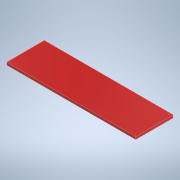
# Autodesk Inventor part: Hanging Platform
Saved by Autodesk Inventor 2021 (Build 250183000, 183)
## iProperties
Created: 2021-02-06
Part Number: Hanging Platform
Material: Rubber, Silicone
Document SubType Name: Modeling
Designer: aidan
Density: 1.25 g/cm^3
Appearance: Red
Author: aidan
Autodesk Inventor part; units mm, degrees
ref_plane "YZ Plane" through (0, 0, 0) normal (1, 0, 0) x (0, 1, 0)
ref_plane "XZ Plane" through (0, 0, 0) normal (0, 1, 0) x (-1, 0, 0)
ref_plane "XY Plane" through (0, 0, 0) normal (0, 0, 1) x (1, 0, 0)
sketch "Sketch1" plane through (0, 0, 0) normal (0, 1, 0) x (-1, 0, 0)
  line L0 (0, 0) -> (-3657.6, 0)
  line L1 (-3657.6, 0) -> (-3657.6, -1066.8)
  line L2 (-3657.6, -1066.8) -> (0, -1066.8)
  line L3 (0, -1066.8) -> (0, 0)
  dimension "d0" = 3657.6
  dimension "d1" = 1066.8
  constraints: 8 end point, 2 parallel, 1 horizontal, 1 perpendicular
  measures "d0" distance of L1.end L2.end
  measures "d1" distance of L0.end L1.end
extrude "Extrusion1" add sketch "Sketch1" along normal blind 76.2
sketch "Sketch2" plane through (0, 76.2, 0) normal (0, 1, 0) x (1, 0, 0)
  circle A0 centre (50.8, 50.8) radius 1.905
  line L0 (0, 0) -> (3657.6, 0) projected
  line L1 (0, 1066.8) -> (0, 0) projected
  line L2 (60.325, 63.6506) -> (60.325, 37.6088) construction
  dimension "d4" = 3.81
  dimension "d5" = 50.8
  dimension "d6" = 50.8
  dimension "d7" = 9.525
  constraints: 2 end point, 1 centre point, 1 vertical
  measures "d4" diameter of A0
  measures "d5" distance from line of L0 A0.centre
  measures "d6" distance from line of L1 A0.centre
  measures "d7" distance from line of L2 A0.centre
revolve "Revolution1" cut sketch "Sketch2" angle 180 about axis through (60.325, 76.2, -63.6506) along (0, 0, 1)
sketch "Sketch3" plane through (0, 76.2, 0) normal (0, 1, 0) x (1, 0, 0)
  circle A0 centre (50.8, 50.8) radius 1.905 projected
  line L0 (50.8, 50.8) -> (3597.275, 50.8) construction
  line L1 (3597.275, 50.8) -> (3597.275, 1016) construction
  line L2 (3597.275, 1016) -> (50.8, 1016) construction
  line L3 (50.8, 1016) -> (50.8, 50.8) construction
  line L4 (3657.6, 1066.8) -> (0, 1066.8) projected
  line L5 (3657.6, 0) -> (3657.6, 1066.8) projected
  point P0 (0, 0)
  dimension "d9" = 50.8
  dimension "d10" = 60.325
  constraints: 8 end point, 3 coincident, 2 parallel, 1 horizontal, 1 perpendicular
  measures "d9" distance between parallel lines of L4 L2
  measures "d10" distance between parallel lines of L5 L1
pattern_sketch "Sketch Driven Pattern1" of "Revolution1" from (60.325, 76.2, -50.8) copies at (50.8, 76.2, -1016) at (3597.275, 76.2, -1016) at (3597.275, 76.2, -50.8)
body "Solid1"
